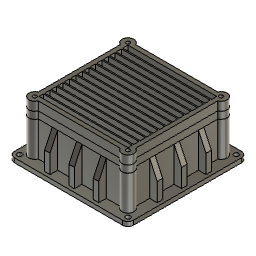
Fan_Mount (Autodesk Fusion 360 design; units mm, degrees)
Autodesk Fusion 360 part; units mm, degrees
note: some values were not read from the file. Set by a fixed rule: which sketch regions a step uses.
sketch "Sketch1" plane through (0, 0, 0) normal (0, 0, 1) x (1, 0, 0)
  line L0 (0, 0) -> (100, 0) construction
  line L1 (100, 0) -> (100, 100) construction
  line L2 (100, 100) -> (0, 100) construction
  line L3 (0, 100) -> (0, 0) construction
  circle A0 centre (0, 100) radius 2.25
  circle A1 centre (100, 100) radius 2.25
  circle A2 centre (100, 0) radius 2.25
  circle A3 centre (0, 0) radius 2.25
  line L4 (-5, 105) -> (105, 105)
  line L5 (105, 105) -> (105, -5)
  line L6 (105, -5) -> (-5, -5)
  line L7 (-5, -5) -> (-5, 105)
  line L8 (50, 105) -> (50, -5) construction
  line L9 (-5, 50) -> (105, 50) construction
  line L10 (14.25, 85.75) -> (85.75, 85.75) construction
  line L11 (85.75, 85.75) -> (85.75, 14.25) construction
  line L12 (85.75, 14.25) -> (14.25, 14.25) construction
  line L13 (14.25, 14.25) -> (14.25, 85.75) construction
  circle A4 centre (85.75, 85.75) radius 1.95
  circle A5 centre (85.75, 14.25) radius 1.95
  circle A6 centre (14.25, 14.25) radius 1.95
  circle A7 centre (14.25, 85.75) radius 1.95
  circle A8 centre (50, 50) radius 46 construction
  line L14 (10, 90) -> (90, 90) construction
  line L15 (90, 90) -> (90, 10) construction
  line L16 (90, 10) -> (10, 10) construction
  line L17 (10, 10) -> (10, 90) construction
  line L18 (27.2844, 90) -> (72.7156, 90)
  line L19 (90, 72.7156) -> (90, 27.2844)
  line L20 (72.7156, 10) -> (27.2844, 10)
  line L21 (10, 27.2844) -> (10, 72.7156)
  arc A9 (27.2844, 90) -> (10, 72.7156) centre (50, 50) ccw
  arc A10 (90, 72.7156) -> (72.7156, 90) centre (50, 50) ccw
  arc A11 (72.7156, 10) -> (90, 27.2844) centre (50, 50) ccw
  arc A12 (10, 27.2844) -> (27.2844, 10) centre (50, 50) ccw
  line L22 (5, 95) -> (95, 95)
  line L23 (95, 95) -> (95, 5)
  line L24 (95, 5) -> (5, 5)
  line L25 (5, 5) -> (5, 95)
  circle A13 centre (14.25, 85.75) radius 4.05
  circle A14 centre (85.75, 85.75) radius 4.05
  circle A15 centre (14.25, 14.25) radius 4.05
  circle A16 centre (85.75, 14.25) radius 4.05
  line L26 (9, 91) -> (91, 91)
  line L27 (91, 91) -> (91, 9)
  line L28 (91, 9) -> (9, 9)
  line L29 (9, 9) -> (9, 91)
  circle A17 centre (93, 93) radius 4.05
  circle A18 centre (93, 93) radius 1.95
  line L30 (93, 93) -> (7, 93) construction
  line L31 (7, 93) -> (7, 7) construction
  line L32 (7, 7) -> (93, 7) construction
  line L33 (93, 7) -> (93, 93) construction
  circle A19 centre (93, 7) radius 1.95
  circle A20 centre (93, 7) radius 4.05
  circle A21 centre (7, 7) radius 4.05
  circle A22 centre (7, 7) radius 1.95
  circle A23 centre (7, 93) radius 4.05
  circle A24 centre (7, 93) radius 1.95
  circle A25 centre (72.7156, 10) radius 4
  arc A26 (12.1235, 95) -> (5, 87.8765) centre (7, 93) ccw
  arc A27 (95, 87.8765) -> (87.8765, 95) centre (93, 93) ccw
  arc A28 (87.8765, 5) -> (95, 12.1235) centre (93, 7) ccw
  arc A29 (5, 12.1235) -> (12.1235, 5) centre (7, 7) ccw
  circle A30 centre (0, 0) radius 4
  circle A31 centre (0, 100) radius 4
  circle A32 centre (100, 100) radius 4
  circle A33 centre (100, 0) radius 4
  line L34 (47.5, 5) -> (52.5, 5)
  line L35 (52.5, 5) -> (52.5, -2)
  line L36 (52.5, -2) -> (47.5, -2)
  line L37 (47.5, -2) -> (47.5, 5)
  line L38 (25, 5) -> (30, 5)
  line L39 (30, 5) -> (30, -2)
  line L40 (30, -2) -> (25, -2)
  line L41 (25, -2) -> (25, 5)
  line L42 (70, 5) -> (75, 5)
  line L43 (75, 5) -> (75, -2)
  line L44 (75, -2) -> (70, -2)
  line L45 (70, -2) -> (70, 5)
  line L46 (25, 95) -> (30, 95)
  line L47 (30, 95) -> (30, 102)
  line L48 (30, 102) -> (25, 102)
  line L49 (25, 102) -> (25, 95)
  line L50 (47.5, 95) -> (52.5, 95)
  line L51 (52.5, 95) -> (52.5, 102)
  line L52 (52.5, 102) -> (47.5, 102)
  line L53 (47.5, 102) -> (47.5, 95)
  line L54 (70, 95) -> (75, 95)
  line L55 (75, 95) -> (75, 102)
  line L56 (75, 102) -> (70, 102)
  line L57 (70, 102) -> (70, 95)
  line L58 (5, 75) -> (-2, 75)
  line L59 (-2, 75) -> (-2, 70)
  line L60 (-2, 70) -> (5, 70)
  line L61 (5, 70) -> (5, 75)
  line L62 (5, 52.5) -> (-2, 52.5)
  line L63 (-2, 52.5) -> (-2, 47.5)
  line L64 (-2, 47.5) -> (5, 47.5)
  line L65 (5, 47.5) -> (5, 52.5)
  line L66 (5, 30) -> (-2, 30)
  line L67 (-2, 30) -> (-2, 25)
  line L68 (-2, 25) -> (5, 25)
  line L69 (5, 25) -> (5, 30)
  line L70 (95, 75) -> (102, 75)
  line L71 (102, 75) -> (102, 70)
  line L72 (102, 70) -> (95, 70)
  line L73 (95, 70) -> (95, 75)
  line L74 (95, 52.5) -> (102, 52.5)
  line L75 (102, 52.5) -> (102, 47.5)
  line L76 (102, 47.5) -> (95, 47.5)
  line L77 (95, 47.5) -> (95, 52.5)
  line L78 (95, 30) -> (102, 30)
  line L79 (102, 30) -> (102, 25)
  line L80 (102, 25) -> (95, 25)
  line L81 (95, 25) -> (95, 30)
  dimension "d1" = 100
  dimension "d2" = 4.5
  dimension "d3" = 110
  dimension "d4" = 3.9
  dimension "d5" = 71.5
  dimension "d6" = 92
  dimension "d7" = 80
  dimension "d8" = 90
  dimension "d11" = 8.1
  dimension "d12" = 82
  dimension "d22" = 86
  dimension "d52" = 8
  dimension "d57" = 8
  dimension "d58" = 5.5
  dimension "d59" = 5
  dimension "d60" = 40
  dimension "d61" = 40
  dimension "d62" = 40
  dimension "d63" = 40
  dimension "d64" = 7
  constraint horizontal L0
  constraint vertical L1
  constraint horizontal L2
  constraint vertical L3
  constraint coincident L0.start L3.end
  constraint equal L2 L3
  constraint coincident L2.end L3.start
  constraint coincident L1.end L2.start
  constraint coincident L0.end L1.start
  constraint equal A0 A3
  constraint equal A0 A1
  constraint equal A1 A2
  constraint horizontal L4
  constraint vertical L5
  constraint horizontal L6
  constraint vertical L7
  constraint midpoint L4 L8.start
  constraint midpoint L6 L8.end
  constraint midpoint L7 L9.start
  constraint midpoint L5 L9.end
  constraint symmetric L0.start L2.end L9
  constraint symmetric L2.end L1.end L8
  constraint equal L4 L7
  constraint horizontal L10
  constraint vertical L11
  constraint horizontal L12
  constraint vertical L13
  constraint symmetric L8 L10.start L10.end
  constraint symmetric L9 L10.start L12.end
  constraint equal L10 L13
  constraint coincident L10.end L11.start
  constraint coincident L11.end L12.start
  constraint coincident L12.end L13.start
  constraint coincident L10.start L13.end
  constraint equal A4 A7
  constraint equal A4 A5
  constraint equal A5 A6
  constraint midpoint L9 A8.centre
  constraint horizontal L14
  constraint vertical L15
  constraint horizontal L16
  constraint vertical L17
  constraint symmetric L8 L14.start L14.end
  constraint symmetric L9 L14.start L16.end
  constraint equal L14 L17
  constraint coincident A8 L18.start
  constraint coincident L14 L18.start
  constraint coincident A8 L18.end
  constraint coincident L14 L18.end
  constraint coincident A8 L19.start
  constraint coincident L15 L19.start
  constraint coincident A8 L19.end
  constraint coincident L15 L19.end
  constraint coincident L16 L20.start
  constraint coincident A8 L20.start
  constraint coincident A8 L20.end
  constraint coincident L16 L20.end
  constraint coincident A8 L21.start
  constraint coincident L17 L21.start
  constraint coincident A8 L21.end
  constraint coincident L17 L21.end
  constraint coincident A8.centre A9.centre
  constraint horizontal L22
  constraint vertical L23
  constraint horizontal L24
  constraint vertical L25
  constraint symmetric L8 L22.start L22.end
  constraint symmetric L9 L22.start L24.end
  constraint equal L22 L25
  constraint concentric A7 A13
  constraint concentric A4 A14
  constraint concentric A6 A15
  constraint concentric A5 A16
  constraint equal A13 A15
  constraint equal A15 A16
  constraint equal A14 A16
  constraint horizontal L26
  constraint vertical L27
  constraint horizontal L28
  constraint vertical L29
  constraint symmetric L8 L26.start L26.end
  constraint symmetric L9 L26.start L28.end
  constraint equal L26 L29
  constraint concentric A17 A18
  constraint equal A14 A17
  constraint equal A4 A18
  constraint horizontal L30
  constraint vertical L31
  constraint horizontal L32
  constraint vertical L33
  constraint coincident A17.centre A18.centre
  constraint symmetric L8 A17.centre L30.end
  constraint symmetric L9 L30.end L31.end
  constraint equal L30 L31
  constraint coincident L32.end L33.start
  constraint concentric A19 A20
  constraint coincident L31.end L32.start
  constraint concentric A21 A22
  constraint coincident L30.end L31.start
  constraint concentric A23 A24
  constraint equal A18 A24
  constraint equal A22 A24
  constraint equal A19 A22
  constraint equal A21 A23
  constraint equal A20 A23
  constraint equal A17 A20
  constraint coincident L20.start A11.start
  constraint coincident L25 A26.end
  constraint coincident L22 A26.start
  constraint coincident L23 A27.start
  constraint coincident L22 A27.end
  constraint coincident L24 A28.start
  constraint coincident L23 A28.end
  constraint coincident L24 A29.end
  constraint coincident L25 A29.start
  constraint concentric A3 A30
  constraint concentric A0 A31
  constraint concentric A1 A32
  constraint concentric A2 A33
  constraint equal A30 A33
  constraint equal A30 A31
  constraint equal A31 A32
  constraint equal A26 A27
  constraint equal A27 A28
  constraint equal A28 A29
  constraint horizontal L34
  constraint vertical L35
  constraint horizontal L36
  constraint vertical L37
  constraint coincident L24 L34.start
  constraint horizontal L38
  constraint vertical L39
  constraint horizontal L40
  constraint vertical L41
  constraint coincident L24 L38.start
  constraint horizontal L42
  constraint vertical L43
  constraint horizontal L44
  constraint vertical L45
  constraint coincident L24 L42.start
  constraint horizontal L46
  constraint vertical L47
  constraint horizontal L48
  constraint vertical L49
  constraint coincident L22 L46.start
  constraint horizontal L50
  constraint vertical L51
  constraint horizontal L52
  constraint vertical L53
  constraint coincident L22 L50.start
  constraint horizontal L54
  constraint vertical L55
  constraint horizontal L56
  constraint vertical L57
  constraint coincident L22 L54.start
  constraint horizontal L58
  constraint vertical L59
  constraint horizontal L60
  constraint vertical L61
  constraint coincident L25 L58.start
  constraint horizontal L62
  constraint vertical L63
  constraint horizontal L64
  constraint vertical L65
  constraint coincident L25 L62.start
  constraint horizontal L66
  constraint vertical L67
  constraint horizontal L68
  constraint vertical L69
  constraint coincident L25 L66.start
  constraint horizontal L70
  constraint vertical L71
  constraint horizontal L72
  constraint vertical L73
  constraint coincident L23 L70.start
  constraint horizontal L74
  constraint vertical L75
  constraint horizontal L76
  constraint vertical L77
  constraint coincident L23 L74.start
  constraint horizontal L78
  constraint vertical L79
  constraint horizontal L80
  constraint vertical L81
  constraint coincident L23 L78.start
  constraint symmetric L8 L47.end L56.end
  constraint symmetric L9 L59.end L66.end
  constraint symmetric L8 L40.end L43.end
  constraint symmetric L9 L71.end L78.end
  constraint equal L48 L52
  constraint equal L52 L56
  constraint equal L56 L71
  constraint equal L71 L75
  constraint equal L75 L79
  constraint equal L44 L79
  constraint equal L36 L44
  constraint equal L36 L40
  constraint equal L40 L67
  constraint equal L63 L67
  constraint equal L59 L63
  constraint symmetric L8 L51.end L52.end
  constraint symmetric L9 L62.end L63.end
  constraint symmetric L9 L74.end L75.end
  constraint symmetric L8 L35.end L36.end
  constraint equal L47 L51
  constraint equal L76 L78
  constraint equal L55 L78
  constraint equal L35 L43
  constraint equal L43 L78
  constraint equal L64 L66
  constraint equal L41 L66
  measures "d1" distance of L0.start L0.end
  measures "d2" diameter of A3
  measures "d3" distance of L5.end L6.end
  measures "d4" diameter of A4
  measures "d5" distance of L11.end L12.end
  measures "d6" diameter of A8
  measures "d7" distance of L15.end L16.end
  measures "d8" distance of L23.end L24.end
  measures "d11" diameter of A14
  measures "d12" distance of L27.end L28.end
  measures "d22" distance of L31.end L32.end
  measures "d52" diameter of A25
  measures "d57" diameter of A32
  measures "d58" radius of A27
  measures "d59" distance of L47.end L48.end
  measures "d60" distance of L47.end L56.end
  measures "d61" distance of L71.end L78.end
  measures "d62" distance of L39.end L44.end
  measures "d63" distance of L59.end L66.end
  measures "d64" distance of L46.start L48.end
extrude "Extrude1" add sketch "Sketch1" along normal blind 4 contours L4 L5 L6 L7 | L18 L19 L20 L21 A9 A10 A11 A12 L26 L27 L28 L29 A17 A20 A21 A23 A25 | L24 L28 A20 A21 A25 L34 L38 L42 | L24 L25 L28 L29 A21 | L28 L29 A21 | L27 L28 A20 | L23 L24 L27 L28 A20 | L25 L29 A21 A23 L61 L65 L69 | L23 L27 A17 A20 L73 L77 L81 | L23 L24 A20 A28 | L23 L24 A20 | L24 L25 A21 | L24 L25 A21 A29 | L22 L25 L26 L29 A23 | L26 L29 A23 | L26 L27 A17 | L22 L23 L26 L27 A17 | L22 L25 A23 | L22 L25 A23 A26 | L22 L26 A17 A23 L46 L50 L54 | L22 L23 A17 A27 | L22 L23 A17 | L24 L42 L43 L44 L45 | L24 L38 L39 L40 L41 | L25 L66 L67 L68 L69 | L23 L78 L79 L80 L81 | L25 L58 L59 L60 L61 | L23 L70 L71 L72 L73 | L24 L34 L35 L36 L37 | L22 L46 L47 L48 L49 | L25 L62 L63 L64 L65 | L22 L54 L55 L56 L57 | L23 L74 L75 L76 L77 | L22 L50 L51 L52 L53 | A13 | A14 | A15 | A16 | A18 | A19 | A22 | A24 | A30 | A31 | A32 | A33 makes body 1
extrude "Extrude4" add sketch "Sketch1" along normal blind 6 contours L18 L19 L20 L21 A9 A10 A11 A12 L26 L27 L28 L29 A17 A20 A21 A23 A25 | L24 L28 A20 A21 A25 L34 L38 L42 | L24 L25 L28 L29 A21 | L28 L29 A21 | L27 L28 A20 | L23 L24 L27 L28 A20 | L25 L29 A21 A23 L61 L65 L69 | L23 L27 A17 A20 L73 L77 L81 | L22 L25 L26 L29 A23 | L26 L29 A23 | L26 L27 A17 | L22 L23 L26 L27 A17 | L22 L26 A17 A23 L46 L50 L54 | A13 | A14 | A15 | A16 | A18 | A19 | A22 | A24 bodies 1
extrude "Extrude5" add sketch "Sketch1" along normal blind 36 contours L24 L28 A20 A21 A25 L34 L38 L42 | L28 A25 | L24 L25 L28 L29 A21 | L23 L24 L27 L28 A20 | L25 L29 A21 A23 L61 L65 L69 | L23 L27 A17 A20 L73 L77 L81 | L22 L25 L26 L29 A23 | L22 L23 L26 L27 A17 | L22 L26 A17 A23 L46 L50 L54 | L24 L42 L43 L44 L45 | L24 L38 L39 L40 L41 | L25 L66 L67 L68 L69 | L23 L78 L79 L80 L81 | L25 L58 L59 L60 L61 | L23 L70 L71 L72 L73 | L24 L34 L35 L36 L37 | L22 L46 L47 L48 L49 | L25 L62 L63 L64 L65 | L22 L54 L55 L56 L57 | L23 L74 L75 L76 L77 | L22 L50 L51 L52 L53 | A18 | A19 | A22 | A24 bodies 1
extrude "Extrude6" add sketch "Sketch1" against normal up to surface (36 mm away) from surface at 36 contours L24 L25 L28 L29 A21 | L23 L24 L27 L28 A20 | L23 L24 A20 A28 | L23 L24 A20 | L24 L25 A21 | L24 L25 A21 A29 | L22 L25 L26 L29 A23 | L22 L23 L26 L27 A17 | L22 L25 A23 | L22 L25 A23 A26 | L22 L23 A17 A27 | L22 L23 A17 bodies 1
extrude "Extrude7" cut sketch "Sketch1" against normal blind 30 from surface at 36 contours A18 | A19 | A22 | A24 bodies 1
sketch "Sketch2" plane through (0, 0, 0) normal (0, 0, 1) x (1, 0, 0)
  circle A0 centre (93, 93) radius 4.05
  circle A1 centre (93, 7) radius 4.05
  circle A2 centre (7, 7) radius 4.05
  circle A3 centre (7, 93) radius 4.05
  circle A4 centre (7, 7) radius 4.05
  circle A5 centre (93, 7) radius 4.05
  circle A6 centre (93, 93) radius 4.05
  circle A7 centre (7, 93) radius 4.05
  line L0 (9, 91) -> (91, 91)
  line L1 (91, 91) -> (91, 9)
  line L2 (91, 9) -> (9, 9)
  line L3 (9, 9) -> (9, 91)
  line L4 (5, 95) -> (95, 95)
  line L5 (95, 95) -> (95, 5)
  line L6 (95, 5) -> (5, 5)
  line L7 (5, 5) -> (5, 95)
  circle A8 centre (93, 7) radius 1.75
  circle A9 centre (93, 93) radius 1.75
  circle A10 centre (7, 93) radius 1.75
  circle A11 centre (7, 7) radius 1.75
  line L8 (9, 86.2) -> (91, 86.2)
  line L9 (91, 86.2) -> (91, 85)
  line L10 (91, 85) -> (9, 85)
  line L11 (9, 85) -> (9, 86.2)
  point P0 (7, 93)
  point P1 (93, 93)
  point P2 (93, 7)
  point P3 (7, 7)
  point P4 (91, 9)
  point P5 (9, 91)
  point P6 (5, 95)
  point P7 (95, 5)
  dimension "d29" = 3.5
  dimension "d30" = 1.2
  dimension "d31" = 4.8
  constraint coincident P0 A3.centre
  constraint coincident A0.centre A6.centre
  constraint coincident A1.centre A5.centre
  constraint coincident A2.centre A4.centre
  constraint equal A2 A4
  constraint equal A1 A5
  constraint equal A0 A6
  constraint equal A3 A7
  constraint horizontal L0
  constraint vertical L1
  constraint horizontal L2
  constraint vertical L3
  constraint coincident P4 L1.end
  constraint coincident P5 L0.start
  constraint horizontal L4
  constraint vertical L5
  constraint horizontal L6
  constraint vertical L7
  constraint coincident P6 L4.start
  constraint coincident P7 L5.end
  constraint concentric A5 A8
  constraint concentric A0 A9
  constraint concentric A3 A10
  constraint concentric A4 A11
  constraint equal A10 A11
  constraint equal A8 A11
  constraint equal A8 A9
  constraint horizontal L8
  constraint vertical L9
  constraint horizontal L10
  constraint vertical L11
  constraint coincident L1 L9.end
  constraint coincident L3 L8.start
  measures "d29" diameter of A9
  measures "d30" distance of L8.start L10.end
  measures "d31" distance of P5 L8.start
extrude "Extrude8" add sketch "Sketch1" sketch "Sketch2" along normal blind 6.5 separate body contours L23 L24 A20 A28 | L24 L25 A21 A29 | L22 L25 A23 A26 | L22 L23 A17 A27 of sketch 2 contours A0 A6 L4 L5 | A0 A6 L0 L1 L4 L5 | A0 A3 A6 A7 L0 L4 | A0 A1 A5 A6 L1 L5 L9 | A3 A7 L4 L7 | A3 A7 L0 L3 L4 L7 | A1 A5 L1 L2 L5 L6 | A1 A5 L5 L6 | A2 A3 A4 A7 L3 L7 L11 | A2 A4 L6 L7 | A2 A4 L2 L3 L6 L7 | A1 A2 A4 A5 L2 L6 start surface through (0, 0, 36) normal (0, 0, 1) makes body 2
extrude "Extrude9" add sketch "Sketch2" along normal blind 1.5 from surface at 36 contours L1 L3 L8 L9 L10 L11 bodies 2
pattern_linear "R-Pattern1" count 13 spacing 6 along (0, -1, 0) of "Extrude9"
extrude "Extrude10" add sketch "Sketch1" sketch "Sketch2" along normal blind 8 separate body contours L23 L24 A20 A28 | L24 L25 A21 A29 | L22 L25 A23 A26 | L22 L23 A17 A27 of sketch 2 contours A0 A6 L4 L5 | A0 A6 L0 L1 L4 L5 | A0 A3 A6 A7 L0 L4 | A0 A1 A5 A6 L1 L5 L9 | A3 A7 L4 L7 | A3 A7 L0 L3 L4 L7 | A1 A5 L1 L2 L5 L6 | A1 A5 L5 L6 | A2 A3 A4 A7 L3 L7 L11 | A2 A4 L6 L7 | A2 A4 L2 L3 L6 L7 | A1 A2 A4 A5 L2 L6 start surface through (0, 0, 42.5) normal (0, 0, 1) makes body 3
extrude "Extrude11" add sketch "Sketch2" along normal up to surface (8 mm away) from surface at 42.5 contours L1 L3 L8 L9 L10 L11 bodies 3
pattern_linear "R-Pattern2" count 13 spacing 6 along (0, -1, 0) of "Extrude11"
extrude "Extrude12" cut sketch "Sketch1" along normal blind 36 contours L20 A11 L28 A25 | L28 A25 bodies 1
fillet "Fillet1" radius 5 4 edges at (-5, -5, 2) (105, -5, 2) (-5, 105, 2) (105, 105, 2) on bodies 1
chamfer "Chamfer1" distance 7 distance2 15 12 edges at (102, 27.5, 36) (102, 50, 36) (102, 72.5, 36) (72.5, 102, 36) (50, 102, 36) (27.5, 102, 36) (-2, 72.5, 36) (-2, 50, 36) (-2, 27.5, 36) (27.5, -2, 36) (50, -2, 36) (72.5, -2, 36) measured on face at (7.6667, 43.3333, 36) measured on face at (7.6667, 43.3333, 36) measured on face at (7.6667, 43.3333, 36) measured on face at (7.6667, 43.3333, 36) measured on face at (7.6667, 43.3333, 36) measured on face at (7.6667, 43.3333, 36) measured on face at (7.6667, 43.3333, 36) measured on face at (7.6667, 43.3333, 36) measured on face at (7.6667, 43.3333, 36) measured on face at (7.6667, 43.3333, 36) measured on face at (7.6667, 43.3333, 36) measured on face at (7.6667, 43.3333, 36) on bodies 1
equation "d11 = 3.9 mm + ( 2 * 2.1 ) * 1 mm"
equation "d20 = 6 mm + 30 mm"
named bodies: "Fan_Mount_Base", "Fan_Mount_Filter", "Fan_Mount_Cover"
